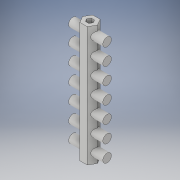
# Autodesk Inventor part: Peg Spinner
Saved by Autodesk Inventor 2019 (Build 230136000, 136)
## iProperties
Created: 2019-01-23
Part Number: Peg Spinner
Material: Generic
Document SubType Name: Modeling
Designer: Ashley
Density: 1 g/cm^3
Appearance: Default
Author: Ashley
Autodesk Inventor part; units mm, degrees
ref_plane "YZ Plane" through (0, 0, 0) normal (1, 0, 0) x (0, 1, 0)
ref_plane "XZ Plane" through (0, 0, 0) normal (0, 1, 0) x (-1, 0, 0)
ref_plane "XY Plane" through (0, 0, 0) normal (0, 0, 1) x (1, 0, 0)
sketch "Outer Diameter Sketch" plane through (0, 0, 0) normal (0, 1, 0) x (-1, 0, 0)
  line L0 (0, -28.0163) -> (0, 28.3344) construction
  line L1 (17.1062, 0) -> (-23.8822, 0) construction
  line L2 (3.4641, -6) -> (6.9282, 0)
  line L3 (6.9282, 0) -> (3.4641, 6)
  line L4 (3.4641, 6) -> (-3.4641, 6)
  line L5 (-3.4641, 6) -> (-6.9282, 0)
  line L6 (-6.9282, 0) -> (-3.4641, -6)
  line L7 (-3.4641, -6) -> (3.4641, -6)
  line L8 (0, -6) -> (0, 6) construction
  line L9 (-6.9282, 0) -> (6.9282, 0) construction
  point P0 (0, 0)
  dimension "d23" = 120
  dimension "d25" = 120
  dimension "d27" = 120
  dimension "d29" = 120
  dimension "d31" = 120
  dimension "d32" = 12
  constraints: 20 end point, 3 equal length, 3 midpoint, 2 horizontal, 2 parallel, 2 point on line, 2 vertical, 1 collinear, 1 perpendicular
  measures "d23" angle of L3 L2
  measures "d25" angle of L4 L3
  measures "d27" angle of L5 L4
  measures "d29" angle of L6 L5
  measures "d31" angle of L7 L6
  measures "d32" distance between parallel lines of L4 L7
extrude "Outer Diameter Extrusion" add sketch "Outer Diameter Sketch" along normal mid plane 112
sketch "Sketch2" plane through (0, 0, 0) normal (1, 0, 0) x (0, 1, 0)
  circle A0 centre (0, 0) radius 4
  line L0 (-56, 0) -> (0, 0) construction
  line L1 (0, 0) -> (56, 0) construction
  circle A1 centre (15.6667, 0) radius 4
  circle A2 centre (31.3333, 0) radius 4
  circle A3 centre (47, 0) radius 4
  circle A4 centre (-15.6667, 0) radius 4
  circle A5 centre (0, 0) radius 4
  circle A6 centre (15.6667, 0) radius 4
  circle A7 centre (31.3333, 0) radius 4
  circle A8 centre (-31.3333, 0) radius 4
  circle A9 centre (-15.6667, 0) radius 4
  circle A10 centre (0, 0) radius 4
  circle A11 centre (15.6667, 0) radius 4
  circle A12 centre (-47, 0) radius 4
  circle A13 centre (-31.3333, 0) radius 4
  circle A14 centre (-15.6667, 0) radius 4
  circle A15 centre (0, 0) radius 4
  dimension "d3" = 8
  dimension "d5" = 112
  dimension "d8" = 15.6667
  dimension "d11" = 15.6667
  constraints: 16 centre point, 16 coincident, 4 end point, 3 horizontal, 1 collinear, 1 point on line, 45 other
  measures "d3" diameter of A0
  measures "d5" distance of L1.end L0.start
  measures "d8" distance of L0.end A1.centre
  measures "d11" distance of L0.end A4.centre
extrude "Extrusion2" add sketch "Sketch2" along normal mid plane 32
sketch "Sketch3" plane through (0, -56, 0) normal (0, -1, 0) x (1, 0, 0)
  line L0 (1.55, -2.6847) -> (-1.55, -2.6847)
  line L1 (-1.55, -2.6847) -> (-3.1, 0)
  line L2 (-3.1, 0) -> (-1.55, 2.6847)
  line L3 (-1.55, 2.6847) -> (1.55, 2.6847)
  line L4 (1.55, 2.6847) -> (3.1, 0)
  line L5 (3.1, 0) -> (1.55, -2.6847)
  line L6 (3.1, 0) -> (-3.1, 0) construction
  line L7 (0, 2.6847) -> (0, -2.6847) construction
  line L8 (10.3659, 0) -> (-11.745, 0) construction
  line L9 (0, -9.4896) -> (0, 9.303) construction
  point P0 (0, 0)
  dimension "d33" = 3.1
  dimension "d34" = 3.1
  dimension "d35" = 120
  dimension "d36" = 3.1
  dimension "d37" = 120
  dimension "d38" = 3.1
  dimension "d39" = 120
  dimension "d40" = 3.1
  dimension "d41" = 120
  constraints: 20 end point, 3 horizontal, 3 midpoint, 2 parallel, 2 vertical, 1 collinear, 1 point on line
  measures "d33" distance of L0.start L0.end
  measures "d34" distance of L0.end L1.end
  measures "d35" angle of L0 L1
  measures "d36" distance of L1.end L2.end
  measures "d37" angle of L1 L2
  measures "d38" distance of L2.end L3.end
  measures "d39" angle of L2 L3
  measures "d40" distance of L3.end L4.end
  measures "d41" angle of L3 L4
extrude "Extrusion3" cut sketch "Sketch3" against normal up to surface (112 mm away)
equation "\"d1\" = outL"
equation "\"d3\" = pegD"
equation "\"d5\" = outL"
equation "\"d14\" = pegL + 2 * outD"
equation "\"d33\" = inhexSL"
equation "\"d34\" = inhexSL"
equation "\"d36\" = inhexSL"
equation "\"d38\" = inhexSL"
equation "\"d40\" = inhexSL"
equation "\"d42\" = pegL + 2 * outD"
equation "\"outD\" = 12"
equation "\"inhexSL\" = 3.1"
equation "\"outL\" = 112"
equation "\"pegL\" = 8"
equation "\"pegD\" = 8"
equation "\"outhexSL\" = 5"
body "Solid1"
